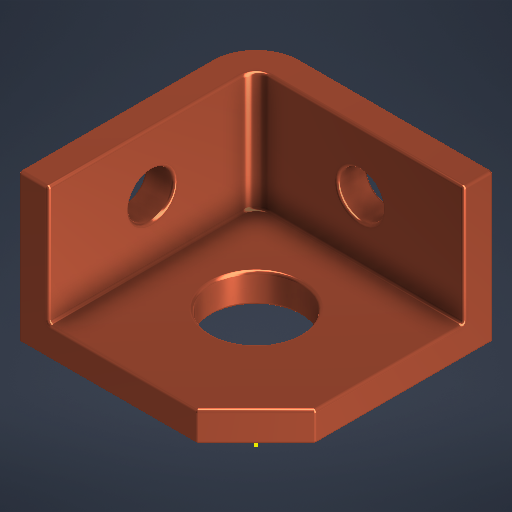
# Autodesk Inventor part: Part3
Saved by Autodesk Inventor 2026.2 (Build 302298000, 298)
## iProperties
Created: 2025-12-08
Part Number: Part3
Material: Steel, Galvanized
Document SubType Name: Modeling
Designer: Thoma
Density: 7.85 g/cm^3
Appearance: Metal 1400F Hot
Author: Thoma
Autodesk Inventor part; units mm, degrees
ref_plane "YZ Plane" through (0, 0, 0) normal (1, 0, 0) x (0, 1, 0)
ref_plane "XZ Plane" through (0, 0, 0) normal (0, 1, 0) x (-1, 0, 0)
ref_plane "XY Plane" through (0, 0, 0) normal (0, 0, 1) x (1, 0, 0)
sketch "Sketch1" plane through (0, 0, 0) normal (0, 1, 0) x (-1, 0, 0)
  line L0 (0, 0) -> (80, 0)
  line L1 (80, 0) -> (80, -80)
  line L2 (80, -80) -> (0, -80)
  line L3 (0, -80) -> (0, 0)
  circle A0 centre (40, -40) radius 15
  line L4 (0, 0) -> (0, -16.4166)
  line L5 (0, -20) -> (20, 0)
  dimension "d0" = 80
  dimension "d1" = 80
  dimension "d2" = 30
  dimension "d3" = 40
  dimension "d4" = 40
  dimension "d5" = 20
  dimension "d6" = 20
  constraints: 12 end point, 3 point on line, 2 parallel, 2 perpendicular, 1 centre point, 1 horizontal
  measures "d0" distance of L0.end L1.end
  measures "d1" distance of L0.start L0.end
  measures "d2" diameter of A0
  measures "d3" distance from line of A0.centre L1
  measures "d4" distance from line of A0.centre L0
  measures "d5" distance of L0.start L5.end
  measures "d6" distance of L5.start L0.start
extrude "Extrusion1" add sketch "Sketch1" along normal blind 10 contours L0 L1 L2 L3 L5
sketch "Sketch2" plane through (0, 10, 0) normal (0, 1, 0) x (1, 0, 0)
  point P0 (0, 0)
sketch "Sketch3" plane through (0, 10, 0) normal (0, 1, 0) x (1, 0, 0)
  line L0 (-80, 80) -> (-80, 0) projected
  line L1 (-80, 70) -> (0, 70)
  line L2 (0, 20) -> (0, 80) projected
  line L3 (0, 80) -> (-80, 80) projected
  line L4 (-80, 0) -> (-20, 0) projected
  line L5 (-70, 80) -> (-70, 0)
  point P0 (0, 0)
  point P1 (-70, 70)
  dimension "d9" = 10
  dimension "d11" = 10
  constraints: 4 end point, 4 point on line, 1 horizontal, 1 perpendicular
  measures "d9" distance of L1.end L2.end
  measures "d11" distance of L5.start L0.start
extrude "Extrusion2" add sketch "Sketch3" along normal blind 40
fillet "Fillet1" radius 5 1 edges at (-70, 30, -70)
fillet "Fillet2" radius 15 1 edges at (-80, 25, -80)
sketch "Sketch4" plane through (0, 10, -70) normal (0, 0, 1) x (1, 0, 0)
  circle A0 centre (-35, 20) radius 7.5
  line L0 (-65, 40) -> (0, 40) projected
  line L1 (0, 0) -> (0, 40) projected
  point P0 (0, -10)
  dimension "d16" = 15
  dimension "d17" = 20
  dimension "d18" = 35
  constraints: 1 centre point
  measures "d16" diameter of A0
  measures "d17" distance from line of A0.centre L0
  measures "d18" distance from line of A0.centre L1
extrude "Extrusion3" cut sketch "Sketch4" against normal blind 10
sketch "Sketch5" plane through (-70, 10, 0) normal (1, 0, 0) x (0, 0, -1)
  circle A0 centre (35, 20) radius 7.5
  line L0 (0, 0) -> (0, 40) projected
  line L1 (0, 40) -> (65, 40) projected
  point P0 (0, -10)
  dimension "d21" = 15
  dimension "d22" = 35
  dimension "d23" = 20
  constraints: 1 centre point
  measures "d21" diameter of A0
  measures "d22" distance from line of A0.centre L0
  measures "d23" distance from line of A0.centre L1
extrude "Extrusion4" cut sketch "Sketch5" against normal blind 10
fillet "Fillet3" radius 1 28 edges at (-32.5, 50, -70) (-70, 50, -32.5) (-75.6066, 50, -75.6066) (-32.5, 50, -80) (-80, 50, -32.5) (-75, 50, 0) (0, 50, -75) (0, 30, -70) (-70, 30, 0) (-70, 10, -32.5) (-68.5355, 10, -68.5355) (-32.5, 10, -70) (0, 0, -50) (0, 25, -80) (0, 10, -45) (0, 5, -20) (-10, 0, -10) (-10, 10, -10) (-20, 5, 0) (-50, 0, 0) (-45, 10, 0) (-80, 25, 0) (-42.5, 30, -70) (-70, 30, -27.5) (-42.5, 30, -80) (-80, 30, -27.5) (-25, 0, -40) (-25, 10, -40)
body "Solid1"
